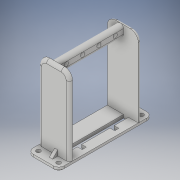
# Autodesk Inventor part: Stewart-Base
Saved by Autodesk Inventor 2018.2 (Build 222227000, 227)
## iProperties
Created: 2018-02-17
Part Number: Stewart-Base
Material: Generisch
Document SubType Name: Modeling
Designer: JochenAlt
Density: 1 g/cm^3
Appearance: Vorgabe
Author: JochenAlt
Autodesk Inventor part; units mm, degrees
ref_plane "YZ Plane" through (0, 0, 0) normal (1, 0, 0) x (0, 1, 0)
ref_plane "XZ Plane" through (0, 0, 0) normal (0, 1, 0) x (-1, 0, 0)
ref_plane "XY Plane" through (0, 0, 0) normal (0, 0, 1) x (1, 0, 0)
sketch "Skizze1" plane through (0, 0, 0) normal (0, 0, 1) x (1, 0, 0)
  line L0 (0, 41.3468) -> (0, -41.3468) construction
  line L1 (-50.7, 0) -> (8.45, 0) construction
  line L2 (-42.25, 19.95) -> (-10, 19.95) construction
  line L3 (-10, 19.95) -> (-10, -19.95) construction
  line L4 (-10, -19.95) -> (-42.25, -19.95) construction
  line L5 (-42.25, -19.95) -> (-42.25, 19.95) construction
  line L6 (-16.3, 19.95) -> (-16.3, -19.95) construction
  line L7 (-18.8, 19.95) -> (-18.8, -19.95) construction
  line L8 (-10, 0.15) -> (-42.25, 0.15) construction
  line L9 (-10, -0.15) -> (-42.25, -0.15) construction
  line L10 (-13.384, 11.05) -> (-16.3, 11.05) construction
  line L11 (-13.384, 9.05) -> (-16.3, 9.05) construction
  line L12 (-10, -9.05) -> (-28.8188, -9.05) construction
  line L13 (-13.384, -11.05) -> (-16.3, -11.05) construction
  line L14 (-13.384, 11.05) -> (-13.384, -11.05) construction
  line L15 (-29.1, 22.25) -> (-29.1, -22.25)
  line L16 (-29.1, 20.25) -> (-10, 20.25)
  line L17 (-29.1, 22.25) -> (-10, 22.25)
  line L18 (-29.1, -20.25) -> (-10, -20.25)
  line L19 (-29.1, -22.25) -> (-10, -22.25)
  line L20 (-10, 22.25) -> (-10, -22.25)
  line L21 (-19.1, 20.25) -> (-19.1, -20.25)
  line L22 (-16, 20.25) -> (-16, -20.25)
  line L23 (-16, 11.35) -> (-13.084, 11.35)
  line L24 (-13.084, 11.35) -> (-13.084, 8.75)
  line L25 (-13.084, 8.75) -> (-16, 8.75)
  line L26 (-16, -8.75) -> (-13.084, -8.75)
  line L27 (-13.084, -8.75) -> (-13.084, -11.35)
  line L28 (-13.084, -11.35) -> (-16, -11.35)
  line L29 (-23.1, 20.25) -> (-23.1, -20.25)
  line L30 (-23.1, 20.25) -> (-23.1, 22.25)
  line L31 (-23.1, -20.25) -> (-23.1, -22.25)
  line L32 (-19.1, -20.25) -> (-19.1, -22.25)
  line L33 (-19.1, 20.25) -> (-19.1, 22.25)
  line L34 (-25.8, -28.85) -> (-13.3, -28.85)
  line L35 (-25.8, 28.85) -> (-13.3, 28.85)
  line L36 (-29.1, -22.25) -> (-29.1, -25.55)
  line L37 (-10, -22.25) -> (-10, -25.55)
  line L38 (-29.1, 22.25) -> (-29.1, 25.55)
  line L39 (-10, 22.25) -> (-10, 25.55)
  arc A0 (-29.1, -25.55) -> (-25.8, -28.85) centre (-25.8, -25.55) ccw
  arc A1 (-13.3, -28.85) -> (-10, -25.55) centre (-13.3, -25.55) ccw
  arc A2 (-10, 25.55) -> (-13.3, 28.85) centre (-13.3, 25.55) ccw
  arc A3 (-25.8, 28.85) -> (-29.1, 25.55) centre (-25.8, 25.55) ccw
  circle A4 centre (-25.8, -25.55) radius 1.3
  circle A5 centre (-13.3, -25.55) radius 1.3
  circle A6 centre (-25.8, 25.55) radius 1.3
  circle A7 centre (-13.3, 25.55) radius 1.3
  point P0 (0, 0)
  point P1 (-16, -15.05)
  point P2 (-16, -5.05)
  point P3 (-16, 5.05)
  point P4 (-16, 15.05)
  dimension "d2" = 6.3
  dimension "d3" = 2.5
  dimension "d5" = 0.3
  dimension "d6" = 8.9
  dimension "d7" = 2
  dimension "d9" = 3.384
  dimension "d10" = 32.25
  dimension "d12" = 2
  dimension "d13" = 0.3
  dimension "d14" = 0.3
  dimension "d15" = 0.3
  dimension "d16" = 0.3
  dimension "d17" = 0.3
  dimension "d18" = 0.3
  dimension "d27" = 4
  dimension "d30" = 4.9
  dimension "d31" = 10
  dimension "d40" = 19.8
  dimension "d41" = 10
  dimension "d43" = 3.3
  dimension "d46" = 10
  dimension "d47" = 2.6
  dimension "d48" = 2
  constraints: 76 end point, 36 point on line, 11 parallel, 10 perpendicular, 8 centre point, 8 horizontal, 8 point on circle, 8 tangent, 8 vertical, 6 equal radius, 4 coincident, 2 symmetric about line, 1 collinear, 9 other
  measures "d2" distance between parallel lines of L3 L6
  measures "d3" distance between parallel lines of L7 L6
  measures "d5" distance between parallel lines of L9 L8
  measures "d6" distance between parallel lines of L10 L2
  measures "d7" distance between parallel lines of L11 L10
  measures "d9" distance between parallel lines of L3 L14
  measures "d10" distance between parallel lines of L5 L3
  measures "d12" distance between parallel lines of L16 L17
  measures "d13" distance between parallel lines of L2 L16
  measures "d14" distance between parallel lines of L7 L21
  measures "d15" distance between parallel lines of L22 L6
  measures "d16" distance between parallel lines of L23 L10
  measures "d17" distance between parallel lines of L11 L25
  measures "d18" distance between parallel lines of L14 L24
  measures "d27" distance between parallel lines of L29 L21
  measures "d30" distance from line of L2 point (-16, 15.05)
  measures "d31" distance of point (-16, 5.05) point (-16, 15.05)
  measures "d40" distance between parallel lines of L8 L2
  measures "d41" distance between parallel lines of L15 L21
  measures "d43" radius of A0
  measures "d46" distance between parallel lines of L0 L3
  measures "d47" diameter of A4
  measures "d48" distance edge to line of A4 L19
extrude "Extrusion1" add sketch "Skizze1" along normal blind 2 contours L17 L30 L16 L15 | L38 A3 L35 A2 L39 L17 | L16 L29 L18 L15 | L17 L33 L16 L30 | L18 L31 L19 L15 | L16 L21 L18 L29 | L17 L20 L16 L33 | L19 L37 A1 L34 A0 L36 | L18 L32 L19 L31 | L18 L20 L19 L32 | L16 L20 L18 L22 L28 L27 L26 L25 L24 L23
extrude "Extrusion2" add sketch "Skizze1" along normal blind 42.9 contours L17 L30 L16 L15 | L17 L33 L16 L30 | L18 L31 L19 L15 | L17 L20 L16 L33 | L18 L32 L19 L31 | L18 L20 L19 L32
extrude "Extrusion4" add sketch "Skizze1" along normal blind 2 from surface at 42.9 contours L17 L30 L16 L15 | L17 L33 L16 L30 | L18 L31 L19 L15 | L16 L21 L18 L29 | L17 L20 L16 L33 | L18 L32 L19 L31 | L18 L20 L19 L32
extrude "Extrusion5" add sketch "Skizze1" along normal blind 5 from surface at 44.9 contours L17 L30 L16 L15 | L17 L33 L16 L30 | L18 L31 L19 L15 | L16 L21 L18 L29 | L17 L20 L16 L33 | L18 L32 L19 L31 | L18 L20 L19 L32
sketch "Skizze2" plane through (-23.1, -22.25, 49.9) normal (-1, 0, 0) x (0, 0, 1)
  line L0 (-49.9, 17.2) -> (0, 17.2) construction
  line L1 (0, 2) -> (0, 42.5) projected
  line L2 (-49.9, 7.2) -> (0, 7.2) construction
  line L3 (-60.36, 22.25) -> (10.06, 22.25) construction
  line L4 (-49.9, 62.64) -> (-49.9, -18.14) construction
  line L5 (-49.9, 27.3) -> (0, 27.3) construction
  line L6 (-49.9, 37.3) -> (0, 37.3) construction
  circle A0 centre (-3.3, 37.3) radius 1.3
  circle A1 centre (-3.3, 27.3) radius 1.3
  circle A2 centre (-3.3, 17.2) radius 1.3
  circle A3 centre (-3.3, 7.2) radius 1.3
  line L7 (-3.3, 37.3) -> (-3.3, 7.2) construction
  line L8 (-49.9, 47.8) -> (-49.9, -3.3) construction
  line L9 (-5, 23.8) -> (-5, 44.4) construction
  point P0 (-49.9, 22.25)
  point P1 (0, 0)
  point P2 (0, 46)
  point P3 (-49.9, -18.14)
  point P4 (-49.3, 46)
  point P5 (-49.3, 0)
  point P6 (-5, 0)
  point P7 (-5, 46)
  point P8 (-7, 42.5)
  point P9 (-7, 2)
  point P10 (-50.3, 44.4)
  point P11 (-50.3, 1.6)
  point P12 (-6, 44.4)
  point P13 (-6.6, 22.2)
  point P14 (-6.6, 23.8)
  point P15 (0, 23.8)
  point P16 (-5, 22.2084)
  point P17 (-5, 1.6)
  point P18 (-49.9, -3.3)
  dimension "d32" = 2.6
  dimension "d34" = 3.7
  constraints: 10 end point, 6 point on line, 4 centre point, 3 equal radius, 3 horizontal, 1 parallel, 1 vertical, 9 other
  measures "d32" diameter of A0
extrude "Extrusion6" cut sketch "Skizze2" against normal blind 20
fillet "Rundung2" radius 5 4 edges at (-29.1, -21.25, 49.9) (-29.1, 21.25, 49.9) (-10, 21.25, 49.9) (-10, -21.25, 49.9)
sketch "Skizze3" plane through (-19.1, 1.15, 0.4) normal (1, 0, 0) x (0, 1, 0)
  line L0 (-23.4, 1.6) -> (-26.7, 1.6) projected
  line L1 (-26.7, 1.6) -> (-23.4, 4.9)
  line L2 (-23.4, 1.6) -> (-23.4, 4.9)
  line L3 (-23.4, 1.6) -> (-26.7, 1.6)
  line L4 (26.4, 1.6) -> (21.1, 4.9)
  line L5 (21.1, 1.6) -> (21.1, 44.5) construction
  line L6 (-23.4, 4.9) -> (21.1, 4.9) construction
  line L7 (-1.15, 59.48) -> (-1.15, -10.38) construction
  line L8 (-41.54, -0.4) -> (39.24, -0.4) construction
  line L9 (21.1, 4.9) -> (21.1, 1.6)
  line L10 (21.1, 1.6) -> (26.4, 1.6)
  point P0 (-1.15, -0.4)
  point P1 (23, 44.3)
  dimension "d49" = 45
  constraints: 14 end point, 2 vertical, 1 collinear, 1 horizontal, 1 parallel, 2 other
  measures "d49" angle of L0 L1
extrude "Extrusion8" add sketch "Skizze3" along normal blind 2
fillet "Rundung3" radius 2 14 edges at (-27.6355, 22.25, 48.4355) (-19.55, 22.25, 49.9) (-11.4645, 22.25, 48.4355) (-10, 22.25, 23.45) (-29.1, 22.25, 23.45) (-11.4645, -22.25, 48.4355) (-19.55, -22.25, 49.9) (-27.6355, -22.25, 48.4355) (-29.1, -22.25, 23.45) (-10, -22.25, 23.45) (-23.1, 0, 49.9) (-19.1, 0, 49.9) (-23.1, 0, 42.9) (-19.1, 0, 42.9)
chamfer "Fase1" distance 0.5 angle 45 8 edges at (-29.1, 0, 0) (-28.1335, -27.8835, 0) (-19.55, -28.85, 0) (-10.9665, -27.8835, 0) (-10, 0, 0) (-10.9665, 27.8835, 0) (-19.55, 28.85, 0) (-28.1335, 27.8835, 0)
equation "\"d14\" = d13"
equation "\"d15\" = d13"
equation "\"d16\" = d13"
equation "\"d17\" = d13"
equation "\"d18\" = d13"
